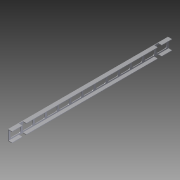
# Autodesk Inventor part: 2.25 U frame front
Saved by Autodesk Inventor 2012 (Build 160160000, 160)
## iProperties
Created: 2013-11-06
Part Number: 2.25 U frame front
Material: Default
Document SubType Name: Modeling
Designer: Bryce
Density: 1 g/cm^3
Author: Bryce
Autodesk Inventor part; units mm, degrees
ref_plane "YZ Plane" through (0, 0, 0) normal (1, 0, 0) x (0, 1, 0)
ref_plane "XZ Plane" through (0, 0, 0) normal (0, 1, 0) x (-1, 0, 0)
ref_plane "XY Plane" through (0, 0, 0) normal (0, 0, 1) x (1, 0, 0)
sketch "Sketch1" plane through (0, 0, 0) normal (0, 0, 1) x (1, 0, 0)
  line L0 (0, 0) -> (22.225, 0)
  line L1 (22.225, 0) -> (22.225, 57.15)
  line L2 (22.225, 57.15) -> (0, 57.15)
  line L3 (0, 57.15) -> (0, 0)
  line L4 (3.175, 3.175) -> (22.225, 3.175)
  line L5 (22.225, 3.175) -> (22.225, 53.975)
  line L6 (22.225, 53.975) -> (3.175, 53.975)
  line L7 (3.175, 53.975) -> (3.175, 3.175)
  dimension "d0" = 3.175
  dimension "d1" = 3.175
  dimension "d2" = 3.175
  dimension "d3" = 57.15
  dimension "d4" = 22.225
  constraints: 16 end point, 4 parallel, 2 horizontal, 2 perpendicular, 1 coincident, 1 point on line
  measures "d0" distance between parallel lines of L0 L4
  measures "d1" distance between parallel lines of L3 L7
  measures "d2" distance between parallel lines of L6 L2
  measures "d3" distance of L2.end L0.start
  measures "d4" distance of L0.start L0.end
extrude "Extrusion1" add sketch "Sketch1" along normal blind 889 contours L3 L2 L1 L6 L7 L4 L0
sketch "Sketch4" plane through (0, 57.15, 0) normal (0, 1, 0) x (1, 0, 0)
  line L0 (22.225, 0) -> (22.225, -889) projected
  line L1 (22.225, 0) -> (0, 0) projected
  line L2 (0, 0) -> (0, -889) projected
  line L3 (22.225, -57.15) -> (3.175, -57.15)
  line L4 (3.175, -57.15) -> (3.175, -79.375)
  line L5 (3.175, -79.375) -> (22.225, -79.375)
  line L6 (22.225, -79.375) -> (22.225, -57.15)
  line L7 (0, -444.5) -> (22.225, -444.5) construction
  line L8 (22.225, -831.85) -> (3.175, -831.85)
  line L9 (3.175, -831.85) -> (3.175, -809.625)
  line L10 (3.175, -809.625) -> (22.225, -809.625)
  line L11 (22.225, -809.625) -> (22.225, -831.85)
  dimension "d33" = 19.05
  dimension "d34" = 22.225
  dimension "d35" = 79.375
  dimension "d36" = 889
  dimension "d37" = 444.5
  constraints: 18 end point, 4 symmetric about line, 2 midpoint, 2 parallel, 2 perpendicular, 1 horizontal, 1 point on line
  measures "d33" distance of L3.start L3.end
  measures "d34" distance of L3.end L4.end
  measures "d35" distance between parallel lines of L1 L5
  measures "d36" distance of L1.end L2.end
  measures "d37" distance between parallel lines of L1 L7
extrude "Extrusion4" cut sketch "Sketch4" against normal through all
sketch "Sketch5" plane through (0, 0, 0) normal (-1, 0, 0) x (0, 0, 1)
  line L0 (889, 0) -> (889, 57.15) projected
  line L1 (0, 57.15) -> (889, 57.15) projected
  line L2 (0, 57.15) -> (0, 0) projected
  line L3 (0, 0) -> (889, 0) projected
  line L4 (879.475, 9.525) -> (65.2323, 9.525) construction
  line L5 (9.525, 9.525) -> (9.525, 47.625) construction
  line L6 (9.525, 47.625) -> (11.9447, 47.625) construction
  line L7 (879.475, 47.625) -> (879.475, 9.525) construction
  arc A0 (11.9447, 47.625) -> (10.7951, 42.4295) centre (85.725, 28.575) ccw construction
  line L8 (72.4144, 47.625) -> (72.4144, 9.525) construction
  line L9 (67.6519, 47.625) -> (67.6519, 9.525) construction
  line L10 (77.1769, 9.525) -> (77.1769, 47.625) construction
  line L11 (4.7625, 47.625) -> (4.7625, 9.525) construction
  arc A1 (65.2323, 9.525) -> (66.3818, 14.7205) centre (-8.5481, 28.575) ccw construction
  line L12 (11.9447, 47.625) -> (17.0392, 47.625) construction
  line L13 (65.2323, 47.625) -> (879.475, 47.625) construction
  line L14 (65.2323, 9.525) -> (60.1377, 9.525) construction
  line L15 (11.9447, 9.525) -> (9.525, 9.525) construction
  arc A2 (17.0392, 47.625) -> (10.7951, 42.4295) centre (17.0392, 41.275) ccw
  arc A3 (66.3818, 42.4295) -> (60.1377, 47.625) centre (60.1377, 41.275) ccw
  arc A4 (60.1377, 9.525) -> (66.3818, 14.7205) centre (60.1377, 15.875) ccw
  arc A5 (10.7951, 14.7205) -> (17.0392, 9.525) centre (17.0392, 15.875) ccw
  arc A6 (10.7951, 42.4295) -> (10.7951, 14.7205) centre (85.725, 28.575) ccw
  line L16 (17.0392, 47.625) -> (60.1377, 47.625)
  line L17 (60.1377, 47.625) -> (65.2323, 47.625) construction
  arc A7 (66.3818, 42.4295) -> (65.2323, 47.625) centre (-8.5481, 28.575) ccw construction
  arc A8 (66.3818, 14.7205) -> (66.3818, 42.4295) centre (-8.5481, 28.575) ccw
  line L18 (60.1377, 9.525) -> (17.0392, 9.525)
  line L19 (17.0392, 9.525) -> (11.9447, 9.525) construction
  arc A9 (10.7951, 14.7205) -> (11.9447, 9.525) centre (85.725, 28.575) ccw construction
  arc A10 (84.6912, 47.625) -> (78.447, 42.4295) centre (84.6912, 41.275) ccw
  arc A11 (134.0338, 42.4295) -> (127.7896, 47.625) centre (127.7896, 41.275) ccw
  arc A12 (127.7896, 9.525) -> (134.0338, 14.7205) centre (127.7896, 15.875) ccw
  arc A13 (78.447, 14.7205) -> (84.6912, 9.525) centre (84.6912, 15.875) ccw
  arc A14 (78.447, 42.4295) -> (78.447, 14.7205) centre (153.3769, 28.575) ccw
  line L20 (84.6912, 47.625) -> (127.7896, 47.625)
  arc A15 (134.0338, 14.7205) -> (134.0338, 42.4295) centre (59.1038, 28.575) ccw
  line L21 (127.7896, 9.525) -> (84.6912, 9.525)
  arc A16 (152.3431, 47.625) -> (146.0989, 42.4295) centre (152.3431, 41.275) ccw
  arc A17 (201.6857, 42.4295) -> (195.4415, 47.625) centre (195.4415, 41.275) ccw
  arc A18 (195.4415, 9.525) -> (201.6857, 14.7205) centre (195.4415, 15.875) ccw
  arc A19 (146.0989, 14.7205) -> (152.3431, 9.525) centre (152.3431, 15.875) ccw
  arc A20 (146.0989, 42.4295) -> (146.0989, 14.7205) centre (221.0288, 28.575) ccw
  line L22 (152.3431, 47.625) -> (195.4415, 47.625)
  arc A21 (201.6857, 14.7205) -> (201.6857, 42.4295) centre (126.7558, 28.575) ccw
  line L23 (195.4415, 9.525) -> (152.3431, 9.525)
  arc A22 (219.995, 47.625) -> (213.7509, 42.4295) centre (219.995, 41.275) ccw
  arc A23 (269.3376, 42.4295) -> (263.0934, 47.625) centre (263.0934, 41.275) ccw
  arc A24 (263.0934, 9.525) -> (269.3376, 14.7205) centre (263.0934, 15.875) ccw
  arc A25 (213.7509, 14.7205) -> (219.995, 9.525) centre (219.995, 15.875) ccw
  arc A26 (213.7509, 42.4295) -> (213.7509, 14.7205) centre (288.6808, 28.575) ccw
  line L24 (219.995, 47.625) -> (263.0934, 47.625)
  arc A27 (269.3376, 14.7205) -> (269.3376, 42.4295) centre (194.4077, 28.575) ccw
  line L25 (263.0934, 9.525) -> (219.995, 9.525)
  arc A28 (287.6469, 47.625) -> (281.4028, 42.4295) centre (287.6469, 41.275) ccw
  arc A29 (336.9895, 42.4295) -> (330.7454, 47.625) centre (330.7454, 41.275) ccw
  arc A30 (330.7454, 9.525) -> (336.9895, 14.7205) centre (330.7454, 15.875) ccw
  arc A31 (281.4028, 14.7205) -> (287.6469, 9.525) centre (287.6469, 15.875) ccw
  arc A32 (281.4028, 42.4295) -> (281.4028, 14.7205) centre (356.3327, 28.575) ccw
  line L26 (287.6469, 47.625) -> (330.7454, 47.625)
  arc A33 (336.9895, 14.7205) -> (336.9895, 42.4295) centre (262.0596, 28.575) ccw
  line L27 (330.7454, 9.525) -> (287.6469, 9.525)
  arc A34 (355.2989, 47.625) -> (349.0547, 42.4295) centre (355.2989, 41.275) ccw
  arc A35 (404.6414, 42.4295) -> (398.3973, 47.625) centre (398.3973, 41.275) ccw
  arc A36 (398.3973, 9.525) -> (404.6414, 14.7205) centre (398.3973, 15.875) ccw
  arc A37 (349.0547, 14.7205) -> (355.2989, 9.525) centre (355.2989, 15.875) ccw
  arc A38 (349.0547, 42.4295) -> (349.0547, 14.7205) centre (423.9846, 28.575) ccw
  line L28 (355.2989, 47.625) -> (398.3973, 47.625)
  arc A39 (404.6414, 14.7205) -> (404.6414, 42.4295) centre (329.7115, 28.575) ccw
  line L29 (398.3973, 9.525) -> (355.2989, 9.525)
  arc A40 (422.9508, 47.625) -> (416.7066, 42.4295) centre (422.9508, 41.275) ccw
  arc A41 (472.2934, 42.4295) -> (466.0492, 47.625) centre (466.0492, 41.275) ccw
  arc A42 (466.0492, 9.525) -> (472.2934, 14.7205) centre (466.0492, 15.875) ccw
  arc A43 (416.7066, 14.7205) -> (422.9508, 9.525) centre (422.9508, 15.875) ccw
  arc A44 (416.7066, 42.4295) -> (416.7066, 14.7205) centre (491.6365, 28.575) ccw
  line L30 (422.9508, 47.625) -> (466.0492, 47.625)
  arc A45 (472.2934, 14.7205) -> (472.2934, 42.4295) centre (397.3635, 28.575) ccw
  line L31 (466.0492, 9.525) -> (422.9508, 9.525)
  arc A46 (490.6027, 47.625) -> (484.3586, 42.4295) centre (490.6027, 41.275) ccw
  arc A47 (539.9453, 42.4295) -> (533.7011, 47.625) centre (533.7011, 41.275) ccw
  arc A48 (533.7011, 9.525) -> (539.9453, 14.7205) centre (533.7011, 15.875) ccw
  arc A49 (484.3586, 14.7205) -> (490.6027, 9.525) centre (490.6027, 15.875) ccw
  arc A50 (484.3586, 42.4295) -> (484.3586, 14.7205) centre (559.2885, 28.575) ccw
  line L32 (490.6027, 47.625) -> (533.7011, 47.625)
  arc A51 (539.9453, 14.7205) -> (539.9453, 42.4295) centre (465.0154, 28.575) ccw
  line L33 (533.7011, 9.525) -> (490.6027, 9.525)
  arc A52 (558.2546, 47.625) -> (552.0105, 42.4295) centre (558.2546, 41.275) ccw
  arc A53 (607.5972, 42.4295) -> (601.3531, 47.625) centre (601.3531, 41.275) ccw
  arc A54 (601.3531, 9.525) -> (607.5972, 14.7205) centre (601.3531, 15.875) ccw
  arc A55 (552.0105, 14.7205) -> (558.2546, 9.525) centre (558.2546, 15.875) ccw
  arc A56 (552.0105, 42.4295) -> (552.0105, 14.7205) centre (626.9404, 28.575) ccw
  line L34 (558.2546, 47.625) -> (601.3531, 47.625)
  arc A57 (607.5972, 14.7205) -> (607.5972, 42.4295) centre (532.6673, 28.575) ccw
  line L35 (601.3531, 9.525) -> (558.2546, 9.525)
  arc A58 (625.9066, 47.625) -> (619.6624, 42.4295) centre (625.9066, 41.275) ccw
  arc A59 (675.2491, 42.4295) -> (669.005, 47.625) centre (669.005, 41.275) ccw
  arc A60 (669.005, 9.525) -> (675.2491, 14.7205) centre (669.005, 15.875) ccw
  arc A61 (619.6624, 14.7205) -> (625.9066, 9.525) centre (625.9066, 15.875) ccw
  arc A62 (619.6624, 42.4295) -> (619.6624, 14.7205) centre (694.5923, 28.575) ccw
  line L36 (625.9066, 47.625) -> (669.005, 47.625)
  arc A63 (675.2491, 14.7205) -> (675.2491, 42.4295) centre (600.3192, 28.575) ccw
  line L37 (669.005, 9.525) -> (625.9066, 9.525)
  arc A64 (693.5585, 47.625) -> (687.3143, 42.4295) centre (693.5585, 41.275) ccw
  arc A65 (742.9011, 42.4295) -> (736.6569, 47.625) centre (736.6569, 41.275) ccw
  arc A66 (736.6569, 9.525) -> (742.9011, 14.7205) centre (736.6569, 15.875) ccw
  arc A67 (687.3143, 14.7205) -> (693.5585, 9.525) centre (693.5585, 15.875) ccw
  arc A68 (687.3143, 42.4295) -> (687.3143, 14.7205) centre (762.2442, 28.575) ccw
  line L38 (693.5585, 47.625) -> (736.6569, 47.625)
  arc A69 (742.9011, 14.7205) -> (742.9011, 42.4295) centre (667.9712, 28.575) ccw
  line L39 (736.6569, 9.525) -> (693.5585, 9.525)
  arc A70 (761.2104, 47.625) -> (754.9662, 42.4295) centre (761.2104, 41.275) ccw
  arc A71 (810.553, 42.4295) -> (804.3088, 47.625) centre (804.3088, 41.275) ccw
  arc A72 (804.3088, 9.525) -> (810.553, 14.7205) centre (804.3088, 15.875) ccw
  arc A73 (754.9662, 14.7205) -> (761.2104, 9.525) centre (761.2104, 15.875) ccw
  arc A74 (754.9662, 42.4295) -> (754.9662, 14.7205) centre (829.8962, 28.575) ccw
  line L40 (761.2104, 47.625) -> (804.3088, 47.625)
  arc A75 (810.553, 14.7205) -> (810.553, 42.4295) centre (735.6231, 28.575) ccw
  line L41 (804.3088, 9.525) -> (761.2104, 9.525)
  arc A76 (828.8623, 47.625) -> (822.6182, 42.4295) centre (828.8623, 41.275) ccw
  arc A77 (878.2049, 42.4295) -> (871.9608, 47.625) centre (871.9608, 41.275) ccw
  arc A78 (871.9608, 9.525) -> (878.2049, 14.7205) centre (871.9608, 15.875) ccw
  arc A79 (822.6182, 14.7205) -> (828.8623, 9.525) centre (828.8623, 15.875) ccw
  arc A80 (822.6182, 42.4295) -> (822.6182, 14.7205) centre (897.5481, 28.575) ccw
  line L42 (828.8623, 47.625) -> (871.9608, 47.625)
  arc A81 (878.2049, 14.7205) -> (878.2049, 42.4295) centre (803.275, 28.575) ccw
  line L43 (871.9608, 9.525) -> (828.8623, 9.525)
  dimension "d40" = 9.525
  dimension "d41" = 9.525
  dimension "d42" = 9.525
  dimension "d43" = 9.525
  dimension "d44" = 76.2
  dimension "d45" = 4.7625
  dimension "d46" = 9.525
  dimension "d47" = 4.7625
  dimension "d48" = 67.6519
  dimension "d49" = 6.35
  dimension "d52" = 67.6519
  constraints: 166 point on circle, 82 centre point, 80 end point, 28 parallel, 23 tangent, 16 point on line, 15 perpendicular, 6 horizontal, 4 equal radius, 2 horizontal alignment, 2 vertical alignment, 264 other
  measures "d40" distance between parallel lines of L2 L5
  measures "d41" distance between parallel lines of L1 L6
  measures "d42" distance between parallel lines of L3 L4
  measures "d43" distance between parallel lines of L0 L7
  measures "d44" radius of A0
  measures "d45" distance between parallel lines of L8 L9
  measures "d46" distance between parallel lines of L10 L9
  measures "d47" distance between parallel lines of L5 L11
  measures "d48" distance between parallel lines of L8 L11
  measures "d49" radius of A2
  measures "d52" distance of A0.centre A14.centre
extrude "Extrusion5" cut sketch "Sketch5" against normal blind 25.4 contours L16 A3 A8 A4 L18 A5 A6 A2 | L20 A11 A15 A12 L21 A13 A14 A10 | L22 A17 A21 A18 L23 A19 A20 A16 | L24 A23 A27 A24 L25 A25 A26 A22 | L26 A29 A33 A30 L27 A31 A32 A28 | L28 A35 A39 A36 L29 A37 A38 A34 | L30 A41 A45 A42 L31 A43 A44 A40 | L32 A47 A51 A48 L33 A49 A50 A46 | L34 A53 A57 A54 L35 A55 A56 A52 | L36 A59 A63 A60 L37 A61 A62 A58 | L38 A65 A69 A66 L39 A67 A68 A64 | L40 A71 A75 A72 L41 A73 A74 A70 | L42 A77 A81 A78 L43 A79 A80 A76
equation "\"d1\" = d0"
equation "\"d2\" = d0"
equation "\"d37\" = 0.5 * d36"
equation "\"d40\" = d41"
equation "\"d42\" = d40"
equation "\"d43\" = d42"
equation "\"d45\" = 0.5 * d46"
equation "\"d46\" = d40"
equation "\"d47\" = 0.5 * d40"
equation "\"d52\" = d48"
body "Solid1"
